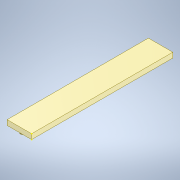
# Autodesk Inventor part: part 2 upper part
Saved by Autodesk Inventor 2021 (Build 250183000, 183)
## iProperties
Created: 2021-07-07
Part Number: part 2 upper part
Material: Generic
Document SubType Name: Modeling
Designer: VK
Density: 1 g/cm^3
Appearance: Nylon 6
Author: VK
Autodesk Inventor part; units mm, degrees
ref_plane "YZ Plane" through (0, 0, 0) normal (1, 0, 0) x (0, 1, 0)
ref_plane "XZ Plane" through (0, 0, 0) normal (0, 1, 0) x (-1, 0, 0)
ref_plane "XY Plane" through (0, 0, 0) normal (0, 0, 1) x (1, 0, 0)
sketch "Sketch1" plane through (0, 0, 0) normal (0, 1, 0) x (-1, 0, 0)
  line L0 (0, 0) -> (24.226, 0)
  line L1 (24.226, 0) -> (24.226, -140)
  line L2 (24.226, -140) -> (0, -140)
  line L3 (0, -140) -> (0, 0)
  dimension "d0" = 24.226
  dimension "d1" = 140
  constraints: 8 end point, 2 parallel, 1 horizontal, 1 perpendicular
  measures "d0" distance of L1.end L2.end
  measures "d1" distance of L0.end L1.end
extrude "Extrusion1" add sketch "Sketch1" along normal blind 5
sketch "Sketch2" plane through (0, 5, 0) normal (0, 1, 0) x (1, 0, 0)
  point P0 (0, 0)
sketch "Sketch3" plane through (0, 0, 0) normal (0, -1, 0) x (1, 0, 0)
  circle A0 centre (-12.113, -2.5) radius 1.5
  point P0 (0, 0)
  dimension "d4" = 3
  constraints: 1 centre point, 1 coincident
  measures "d4" diameter of A0
extrude "Extrusion2" add sketch "Sketch3" along normal blind 2
sketch "Sketch4" plane through (0, 0, 0) normal (0, -1, 0) x (1, 0, 0)
  point P0 (0, 0)
sketch "Sketch5" plane through (-12.113, -2, -2.5) normal (0, -1, 0) x (1, 0, 0)
  line L0 (-0.5, 1.5) -> (0.5, 1.5)
  line L1 (0.5, 1.5) -> (0.5, -1.5)
  line L2 (0.5, -1.5) -> (-0.5, -1.5)
  line L3 (-0.5, -1.5) -> (-0.5, 1.5)
  line L4 (-0.5, 1.5) -> (0.5, -1.5) construction
  line L5 (0.5, 1.5) -> (-0.5, -1.5) construction
  point P0 (12.113, 2.5)
  point P1 (0, 0)
  dimension "d7" = 1
  constraints: 12 end point, 2 midpoint, 2 parallel, 1 horizontal, 1 perpendicular
  measures "d7" distance of L1.end L2.end
extrude "Extrusion3" cut sketch "Sketch5" against normal blind 1.5
pattern_linear "Rectangular Pattern1" count 2 spacing 135 along (0, 0, -1) of "Extrusion2", "Extrusion3"
body "Solid1"
